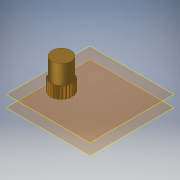
# Autodesk Inventor part: servo_spine
Saved by Autodesk Inventor 2018 (Build 220112000, 112)
## iProperties
Created: 2017-10-09
Part Number: servo_spine
Material: Brass, Soft Yellow
Document SubType Name: Modeling
Designer: liamg
Density: 8.47 g/cm^3
Appearance: Brass - Satin
Author: liamg
Autodesk Inventor part; units mm, degrees
ref_plane "YZ Plane" through (0, 0, 0) normal (1, 0, 0) x (0, 1, 0)
ref_plane "XZ Plane" through (0, 0, 0) normal (0, 1, 0) x (-1, 0, 0)
ref_plane "XY Plane" through (0, 0, 0) normal (0, 0, 1) x (1, 0, 0)
ref_plane "Work Plane6" through (-21.8665, 24.3353, 26.2725) normal (0, 1, 0) x (-1, 0, 0)
sketch "Sketch1" plane through (-21.8665, 24.3353, 26.2725) normal (0, 1, 0) x (-1, 0, 0)
  line L0 (7.495, -2.8448) -> (7.8208, -2.519) projected
  line L1 (7.8208, -2.519) -> (7.8323, -2.5175) projected
  line L2 (7.8323, -2.5175) -> (8.2313, -2.7479) projected
  line L3 (8.2313, -2.7479) -> (8.4616, -2.3489) projected
  line L4 (8.4616, -2.3489) -> (8.4724, -2.3444) projected
  line L5 (8.4724, -2.3444) -> (8.9174, -2.4637) projected
  line L6 (8.9174, -2.4637) -> (9.0366, -2.0186) projected
  line L7 (9.0366, -2.0186) -> (9.0459, -2.0116) projected
  line L8 (9.0459, -2.0116) -> (9.5066, -2.0116) projected
  line L9 (9.5066, -2.0116) -> (9.5066, -1.5509) projected
  line L10 (9.5066, -1.5509) -> (9.5136, -1.5416) projected
  line L11 (9.5136, -1.5416) -> (9.9587, -1.4224) projected
  line L12 (9.9587, -1.4224) -> (9.8394, -0.9774) projected
  line L13 (9.8394, -0.9774) -> (9.8439, -0.9666) projected
  line L14 (9.8439, -0.9666) -> (10.2429, -0.7363) projected
  line L15 (10.2429, -0.7363) -> (10.0125, -0.3373) projected
  line L16 (10.0125, -0.3373) -> (10.014, -0.3258) projected
  line L17 (10.014, -0.3258) -> (10.3398, 0) projected
  line L18 (10.3398, 0) -> (10.014, 0.3258) projected
  line L19 (10.014, 0.3258) -> (10.0125, 0.3373) projected
  line L20 (10.0125, 0.3373) -> (10.2429, 0.7363) projected
  line L21 (10.2429, 0.7363) -> (9.8439, 0.9666) projected
  line L22 (9.8439, 0.9666) -> (9.8394, 0.9774) projected
  line L23 (9.8394, 0.9774) -> (9.9587, 1.4224) projected
  line L24 (9.9587, 1.4224) -> (9.5136, 1.5416) projected
  line L25 (9.5136, 1.5416) -> (9.5066, 1.5509) projected
  line L26 (9.5066, 1.5509) -> (9.5066, 2.0116) projected
  line L27 (9.5066, 2.0116) -> (9.0459, 2.0116) projected
  line L28 (9.0459, 2.0116) -> (9.0366, 2.0186) projected
  line L29 (9.0366, 2.0186) -> (8.9174, 2.4637) projected
  line L30 (8.9174, 2.4637) -> (8.4724, 2.3444) projected
  line L31 (8.4724, 2.3444) -> (8.4616, 2.3489) projected
  line L32 (8.4616, 2.3489) -> (8.2313, 2.7479) projected
  line L33 (8.2313, 2.7479) -> (7.8323, 2.5175) projected
  line L34 (7.8323, 2.5175) -> (7.8208, 2.519) projected
  line L35 (7.8208, 2.519) -> (7.495, 2.8448) projected
  line L36 (7.495, 2.8448) -> (7.1692, 2.519) projected
  line L37 (7.1692, 2.519) -> (7.1577, 2.5175) projected
  line L38 (7.1577, 2.5175) -> (6.7587, 2.7479) projected
  line L39 (6.7587, 2.7479) -> (6.5284, 2.3489) projected
  line L40 (6.5284, 2.3489) -> (6.5176, 2.3444) projected
  line L41 (6.5176, 2.3444) -> (6.0726, 2.4637) projected
  line L42 (6.0726, 2.4637) -> (5.9534, 2.0186) projected
  line L43 (5.9534, 2.0186) -> (5.9441, 2.0116) projected
  line L44 (5.9441, 2.0116) -> (5.4834, 2.0116) projected
  line L45 (5.4834, 2.0116) -> (5.4834, 1.5509) projected
  line L46 (5.4834, 1.5509) -> (5.4764, 1.5416) projected
  line L47 (5.4764, 1.5416) -> (5.0313, 1.4224) projected
  line L48 (5.0313, 1.4224) -> (5.1506, 0.9774) projected
  line L49 (5.1506, 0.9774) -> (5.1461, 0.9666) projected
  line L50 (5.1461, 0.9666) -> (4.7471, 0.7363) projected
  line L51 (4.7471, 0.7363) -> (4.9775, 0.3373) projected
  line L52 (4.9775, 0.3373) -> (4.976, 0.3258) projected
  line L53 (4.976, 0.3258) -> (4.6502, 0) projected
  line L54 (4.6502, 0) -> (4.976, -0.3258) projected
  line L55 (4.976, -0.3258) -> (4.9775, -0.3373) projected
  line L56 (4.9775, -0.3373) -> (4.7471, -0.7363) projected
  line L57 (4.7471, -0.7363) -> (5.1461, -0.9666) projected
  line L58 (5.1461, -0.9666) -> (5.1506, -0.9774) projected
  line L59 (5.1506, -0.9774) -> (5.0313, -1.4224) projected
  line L60 (5.0313, -1.4224) -> (5.4764, -1.5416) projected
  line L61 (5.4764, -1.5416) -> (5.4834, -1.5509) projected
  line L62 (5.4834, -1.5509) -> (5.4834, -2.0116) projected
  line L63 (5.4834, -2.0116) -> (5.9441, -2.0116) projected
  line L64 (5.9441, -2.0116) -> (5.9534, -2.0186) projected
  line L65 (5.9534, -2.0186) -> (6.0726, -2.4637) projected
  line L66 (6.0726, -2.4637) -> (6.5176, -2.3444) projected
  line L67 (6.5176, -2.3444) -> (6.5284, -2.3489) projected
  line L68 (6.5284, -2.3489) -> (6.7587, -2.7479) projected
  line L69 (6.7587, -2.7479) -> (7.1577, -2.5175) projected
  line L70 (7.1577, -2.5175) -> (7.1692, -2.519) projected
  line L71 (7.1692, -2.519) -> (7.495, -2.8448) projected
  circle A0 centre (7.495, 0) radius 1.25 projected
  point P0 (-21.8665, -26.2725)
extrude "Extrusion1" add sketch "Sketch1" along normal blind 3
ref_plane "Work Plane5" through (-21.8665, 27.3353, 26.2725) normal (0, 1, 0) x (1, 0, 0)
sketch "Sketch4" plane through (-21.8665, 27.3353, 26.2725) normal (0, 1, 0) x (1, 0, 0)
  circle A0 centre (-7.495, 0) radius 1.25 construction
  circle A1 centre (-7.495, 0) radius 2.5
  point P0 (21.8665, 26.2725)
  constraints: 1 centre point, 1 coincident
extrude "Extrusion2" add sketch "Sketch4" along normal blind 5
body "Solid1"
